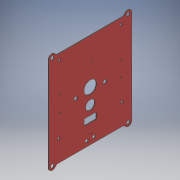
# Autodesk Inventor part: +XPanel_PCB
Saved by Autodesk Inventor 2018 (Build 220112000, 112)
## iProperties
Created: 2018-10-25
Part Number: +XPanel_PCB
Material: Epoxy Resin
Document SubType Name: Modeling
Designer: Bradley
Density: 1.14 g/cm^3
Appearance: Smooth - Dark Gray
Author: Bradley
Autodesk Inventor part; units mm, degrees
ref_plane "YZ Plane" through (0, 0, 0) normal (1, 0, 0) x (0, 1, 0)
ref_plane "XZ Plane" through (0, 0, 0) normal (0, 1, 0) x (-1, 0, 0)
ref_plane "XY Plane" through (0, 0, 0) normal (0, 0, 1) x (1, 0, 0)
sketch "Sketch1" plane through (0, 0, 0) normal (1, 0, 0) x (0, 1, 0)
  line L0 (36.5, -45) -> (-36.5, -45) construction
  line L1 (-36.5, -45) -> (-36.5, 45) construction
  line L2 (-36.5, 45) -> (36.5, 45) construction
  line L3 (36.5, 45) -> (36.5, -45) construction
  line L4 (36.5, -45) -> (-36.5, 45) construction
  line L5 (-36.5, -45) -> (36.5, 45) construction
  line L6 (-14, 0) -> (14, 0) construction
  line L7 (-40, -45) -> (-40, 45)
  arc A0 (-34.0251, 47.4749) -> (-40, 45) centre (-36.5, 45) ccw
  line L8 (-34.0251, 47.4749) -> (-32.3431, 45.7929)
  arc A1 (-32.3431, 45.7929) -> (-31.636, 45.5) centre (-31.636, 46.5) ccw
  line L9 (-31.636, 45.5) -> (31.636, 45.5)
  arc A2 (31.636, 45.5) -> (32.3431, 45.7929) centre (31.636, 46.5) ccw
  line L10 (32.3431, 45.7929) -> (34.0251, 47.4749)
  arc A3 (40, 45) -> (34.0251, 47.4749) centre (36.5, 45) ccw
  line L11 (40, 45) -> (40, -45)
  arc A4 (34.0251, -47.4749) -> (40, -45) centre (36.5, -45) ccw
  line L12 (34.0251, -47.4749) -> (32.3431, -45.7929)
  arc A5 (32.3431, -45.7929) -> (31.636, -45.5) centre (31.636, -46.5) ccw
  line L13 (31.636, -45.5) -> (-31.636, -45.5)
  arc A6 (-31.636, -45.5) -> (-32.3431, -45.7929) centre (-31.636, -46.5) ccw
  line L14 (-32.3431, -45.7929) -> (-34.0251, -47.4749)
  arc A7 (-40, -45) -> (-34.0251, -47.4749) centre (-36.5, -45) ccw
  point P0 (0, 0)
  point P1 (0, 0)
  dimension "d0" = 73
  dimension "d1" = 90
  dimension "d2" = 28
  dimension "d3" = 80
  dimension "d4" = 91
  dimension "d5" = 1
  constraints: 30 end point, 16 point on circle, 16 tangent, 8 centre point, 7 perpendicular, 4 coincident, 4 equal radius, 4 midpoint, 4 parallel, 2 horizontal, 1 vertical
  measures "d0" distance of L1.end L2.end
  measures "d1" distance of L0.end L1.end
  measures "d2" distance of L6.start L6.end
  measures "d3" distance between parallel lines of L11 L7
  measures "d4" distance between parallel lines of L13 L9
  measures "d5" radius of A1
extrude "Extrusion1" add sketch "Sketch1" along normal mid plane 0.6
sketch "Sketch2" plane through (0.3, 0, 0) normal (1, 0, 0) x (0, 0, -1)
  point P0 (0, 0)
  point P1 (-45, -36.5)
  point P2 (-45, 36.5)
  point P3 (0, 14)
  point P4 (0, -14)
  point P5 (45, -36.5)
  point P6 (45, 36.5)
hole "Hole1" at (0.3, -36.5, 45) at (0.3, 36.5, 45) at (0.3, 14, 0) at (0.3, -14, 0) at (0.3, -36.5, -45) at (0.3, 36.5, -45) direction (-1, 0, 0) diameter 3.3 end through all clearance for "Flat Head Machine Screw" size "M3" standard "Ansi Metric M Profile"
sketch "Sketch3" plane through (0.3, 0, 0) normal (1, 0, 0) x (0, 0, -1)
  circle A0 centre (-2.5, 0) radius 6
  circle A1 centre (12.35, 0) radius 4.5
  line L0 (26, -6) -> (22, -6)
  line L1 (21, -5) -> (21, 5)
  line L2 (22, 6) -> (26, 6)
  line L3 (27, 5) -> (27, -5)
  line L4 (27, -6) -> (21, 6) construction
  line L5 (21, -6) -> (27, 6) construction
  arc A2 (21, -5) -> (22, -6) centre (22, -5) ccw
  arc A3 (26, -6) -> (27, -5) centre (26, -5) ccw
  arc A4 (27, 5) -> (26, 6) centre (26, 5) ccw
  arc A5 (22, 6) -> (21, 5) centre (22, 5) ccw
  point P0 (0, 0)
  point P1 (24, 0)
  point P2 (24, 0)
  dimension "d15" = 2.5
  dimension "d16" = 12
  dimension "d17" = 14.85
  dimension "d18" = 9
  dimension "d84" = 24
  dimension "d85" = 12
  dimension "d86" = 6
  dimension "d87" = 1
  constraints: 12 end point, 8 point on circle, 8 point on line, 8 tangent, 6 centre point, 3 equal radius, 3 horizontal alignment, 3 midpoint, 2 parallel, 1 horizontal, 1 perpendicular
  measures "d15" distance of point (0, 0) A0.centre
  measures "d16" diameter of A0
  measures "d17" distance of A1.centre A0.centre
  measures "d18" diameter of A1
  measures "d84" distance of point (0, 0) point (24, 0)
  measures "d85" distance of L5.start L4.end
  measures "d86" distance of L4.start L5.start
  measures "d87" radius of A2
extrude "Extrusion2" cut sketch "Sketch3" against normal through all
sketch "Sketch4" plane through (0.3, 0, 0) normal (1, 0, 0) x (0, 0, -1)
  line L0 (37, -40) -> (38, -40) construction
  line L1 (38, -40) -> (38, 40) construction
  line L2 (38, 40) -> (37, 40) construction
  line L3 (37, 40) -> (37, -40) construction
  line L4 (-11, -40) -> (-10, -40) construction
  line L5 (-10, -40) -> (-10, 40) construction
  line L6 (-10, 40) -> (-11, 40) construction
  line L7 (-11, 40) -> (-11, -40) construction
  circle A0 centre (12.35, 0) radius 4.5 projected
  circle A1 centre (-2.5, 0) radius 6 projected
  circle A2 centre (45, -36.5) radius 1.65 projected
  circle A3 centre (0, 14) radius 1.65 projected
  circle A4 centre (-45, -36.5) radius 1.65 projected
  circle A5 centre (-45, 36.5) radius 1.65 projected
  circle A6 centre (0, -14) radius 1.65 projected
  circle A7 centre (45, 36.5) radius 1.65 projected
  line L8 (-45, -40) -> (45, -40) projected
  arc A8 (45, -40) -> (47.4749, -34.0251) centre (45, -36.5) ccw projected
  line L9 (47.4749, -34.0251) -> (45.7929, -32.3431) projected
  arc A9 (45.5, -31.636) -> (45.7929, -32.3431) centre (46.5, -31.636) ccw projected
  line L10 (45.5, -31.636) -> (45.5, 31.636) projected
  arc A10 (45.7929, 32.3431) -> (45.5, 31.636) centre (46.5, 31.636) ccw projected
  line L11 (45.7929, 32.3431) -> (47.4749, 34.0251) projected
  arc A11 (47.4749, 34.0251) -> (45, 40) centre (45, 36.5) ccw projected
  line L12 (45, 40) -> (-45, 40) projected
  arc A12 (-45, 40) -> (-47.4749, 34.0251) centre (-45, 36.5) ccw projected
  line L13 (-47.4749, 34.0251) -> (-45.7929, 32.3431) projected
  arc A13 (-45.5, 31.636) -> (-45.7929, 32.3431) centre (-46.5, 31.636) ccw projected
  line L14 (-45.5, 31.636) -> (-45.5, -31.636) projected
  arc A14 (-45.7929, -32.3431) -> (-45.5, -31.636) centre (-46.5, -31.636) ccw projected
  line L15 (-45.7929, -32.3431) -> (-47.4749, -34.0251) projected
  arc A15 (-47.4749, -34.0251) -> (-45, -40) centre (-45, -36.5) ccw projected
  line L16 (-20, -40) -> (-19, -40) construction
  line L17 (-19, -40) -> (-19, 40) construction
  line L18 (-20, 40) -> (-20, -40) construction
  line L19 (-19, 40) -> (-20, 40) construction
  line L20 (28, -40) -> (29, -40) construction
  line L21 (29, -40) -> (29, 40) construction
  line L22 (29, 40) -> (28, 40) construction
  line L23 (28, 40) -> (28, -40) construction
  line L24 (-29, -40) -> (-28, -40) construction
  line L25 (-28, -40) -> (-28, 40) construction
  line L26 (-29, 40) -> (-29, -40) construction
  line L27 (-28, 40) -> (-29, 40) construction
  line L28 (19, -40) -> (20, -40) construction
  line L29 (20, -40) -> (20, 40) construction
  line L30 (20, 40) -> (19, 40) construction
  line L31 (19, 40) -> (19, -40) construction
  line L32 (-38, -40) -> (-37, -40) construction
  line L33 (-37, -40) -> (-37, 40) construction
  line L34 (-38, 40) -> (-38, -40) construction
  line L35 (-37, 40) -> (-38, 40) construction
  line L36 (10, -40) -> (11, -40) construction
  line L37 (11, -40) -> (11, 40) construction
  line L38 (11, 40) -> (10, 40) construction
  line L39 (10, 40) -> (10, -40) construction
  line L40 (-10, 0) -> (10, 0) construction
  line L41 (36, -1) -> (36, 1) construction
  circle A16 centre (36, -1) radius 0.75 construction
  circle A17 centre (36, 1) radius 0.75 construction
  circle A18 centre (36, -1) radius 0.35
  circle A19 centre (36, 1) radius 0.35
  line L42 (-38, -13) -> (-12, -13) construction
  line L43 (-12, -13) -> (-12, 13) construction
  line L44 (-12, 13) -> (-38, 13) construction
  line L45 (-38, 13) -> (-38, -13) construction
  circle A20 centre (-23.25, 1.75) radius 0.475
  line L46 (40.5, -3.5) -> (40.5, 3.5) construction
  circle A21 centre (40.5, -3.5) radius 2.25 construction
  circle A22 centre (40.5, 3.5) radius 2.25 construction
  circle A23 centre (28.65, -7) radius 7 construction
  circle A24 centre (21.3666, -25) radius 7 construction
  circle A25 centre (-35.4038, -25) radius 7 construction
  line L47 (35.1389, -9.6256) -> (27.8556, -27.6256) construction
  line L48 (21.3666, -32) -> (-35.4038, -32) construction
  circle A26 centre (25, -30.3897) radius 1 construction
  line L49 (21.3666, -25) -> (25, -30.3897) construction
  arc A27 (21.3666, -32) -> (27.8556, -27.6256) centre (21.3666, -25) ccw construction
  arc A28 (-42.4038, -25) -> (-35.4038, -32) centre (-35.4038, -25) ccw construction
  line L50 (-35.4038, -25) -> (-40, -29.5962) construction
  circle A29 centre (-40, -29.5962) radius 1 construction
  line L51 (35.65, -7) -> (35.65, -1.6633) construction
  line L52 (-42.4038, -25) -> (-42.4038, 0) construction
  line L53 (-45.5, 0) -> (45.5, 0) construction
  line L54 (21.3666, 25) -> (25, 30.3897) construction
  line L55 (-35.4038, 25) -> (-40, 29.5962) construction
  point P0 (36, 0)
  point P1 (0, 0)
  point P2 (-12, 0)
  point P3 (-25, -13)
  point P4 (-38, 0)
  point P5 (-25, 0)
  point P6 (40.5, 0)
  point P7 (25.2795, -30.8043)
  point P8 (-40.3536, -29.9497)
  dimension "d35" = 1.5
  dimension "d25" = 9
  dimension "d30" = 21
  dimension "d31" = 1
  dimension "d34" = 2
  dimension "d38" = 0.7
  dimension "d45" = 26
  dimension "d46" = 12
  dimension "d48" = 0.95
  dimension "d73" = 4.5
  dimension "d74" = 7
  dimension "d75" = 4.5
  dimension "d76" = 40.5
  dimension "d88" = 1.75
  dimension "d89" = 1.75
  dimension "d90" = 14
  dimension "d91" = 7
  dimension "d92" = 7.35
  dimension "d93" = 2
  dimension "d94" = 6.5
  dimension "d96" = 22.03
  dimension "d97" = 32
  dimension "d98" = 40
  dimension "d99" = 25
  constraints: 96 end point, 13 centre point, 12 point on circle, 11 coincident, 10 midpoint, 7 parallel, 7 tangent, 6 point on line, 6 symmetric about line, 5 equal radius, 5 horizontal, 5 horizontal alignment, 3 collinear, 3 equal length, 3 perpendicular, 3 vertical, 1 concentric, 1 vertical alignment, 52 other
  measures "d25" distance of L4.start L16.start
  measures "d30" distance between parallel lines of L37 L5
  measures "d31" distance between parallel lines of L1 L3
  measures "d34" distance of L41.start L41.end
  measures "d38" diameter of A18
  measures "d45" distance of L44.end L43.end
  measures "d46" distance from line of point (0, 0) L43
  measures "d48" diameter of A20
  measures "d73" distance between parallel lines of L46 L41
  measures "d74" distance of L46.start L46.end
  measures "d75" diameter of A21
  measures "d76" distance from line of point (0, 0) L46
  measures "d88" horizontal distance of A20.centre point (-25, 0)
  measures "d89" horizontal distance of A20.centre point (-25, 0)
  measures "d90" diameter of A23
  measures "d91" vertical distance of point (36, 0) A23.centre
  measures "d92" horizontal distance of point (36, 0) A23.centre
  measures "d93" diameter of A26
  measures "d94" distance of L49.start L49.end
  measures "d97" distance from line of A1.centre L48
  measures "d98" horizontal distance of point (0, 0) point (-40, -29.596)
  measures "d99" horizontal distance of point (0, 0) point (25, -30.39)
extrude "Extrusion3" cut sketch "Sketch4" against normal through all contours A18 | A19 | A20
hole "Hole4" at (0.3, -3.5, -40.5) at (0.3, 3.5, -40.5) direction (-1, 0, 0) diameter 3 end through all
hole "Hole5" at (0.3, -30.3897, -25) at (0.3, -29.5962, 40) at (0.3, 30.3897, -25) at (0.3, 29.5962, 40) direction (-1, 0, 0) diameter 2.2 end through all
sketch "Sketch5" plane through (0.3, 0, 0) normal (1, 0, 0) x (0, 0, -1)
  circle A0 centre (25, 30.3897) radius 1.1 projected
  circle A1 centre (25, -30.3897) radius 1.1 projected
  circle A2 centre (-40, -29.5962) radius 1.1 projected
  circle A3 centre (-40, 29.5962) radius 1.1 projected
  circle A4 centre (40.5, -3.5) radius 1.5 projected
  circle A5 centre (40.5, 3.5) radius 1.5 projected
  circle A6 centre (36, -1) radius 0.35 projected
  circle A7 centre (-23.25, 1.75) radius 0.475 projected
  circle A8 centre (36, 1) radius 0.35 projected
  circle A9 centre (12.35, 0) radius 4.5 projected
  circle A10 centre (-2.5, 0) radius 6 projected
  arc A11 (26, -6) -> (27, -5) centre (26, -5) ccw projected
  line L0 (26, -6) -> (22, -6) projected
  arc A12 (21, -5) -> (22, -6) centre (22, -5) ccw projected
  line L1 (21, -5) -> (21, 5) projected
  arc A13 (22, 6) -> (21, 5) centre (22, 5) ccw projected
  line L2 (22, 6) -> (26, 6) projected
  arc A14 (27, 5) -> (26, 6) centre (26, 5) ccw projected
  line L3 (27, 5) -> (27, -5) projected
  circle A15 centre (45, -36.5) radius 1.65 projected
  circle A16 centre (0, 14) radius 1.65 projected
  circle A17 centre (-45, -36.5) radius 1.65 projected
  circle A18 centre (-45, 36.5) radius 1.65 projected
  circle A19 centre (0, -14) radius 1.65 projected
  circle A20 centre (45, 36.5) radius 1.65 projected
  line L4 (-45, -40) -> (45, -40) projected
  arc A21 (45, -40) -> (47.4749, -34.0251) centre (45, -36.5) ccw projected
  line L5 (47.4749, -34.0251) -> (45.7929, -32.3431) projected
  arc A22 (45.5, -31.636) -> (45.7929, -32.3431) centre (46.5, -31.636) ccw projected
  line L6 (45.5, -31.636) -> (45.5, 31.636) projected
  arc A23 (45.7929, 32.3431) -> (45.5, 31.636) centre (46.5, 31.636) ccw projected
  line L7 (45.7929, 32.3431) -> (47.4749, 34.0251) projected
  arc A24 (47.4749, 34.0251) -> (45, 40) centre (45, 36.5) ccw projected
  line L8 (45, 40) -> (-45, 40) projected
  arc A25 (-45, 40) -> (-47.4749, 34.0251) centre (-45, 36.5) ccw projected
  line L9 (-47.4749, 34.0251) -> (-45.7929, 32.3431) projected
  arc A26 (-45.5, 31.636) -> (-45.7929, 32.3431) centre (-46.5, 31.636) ccw projected
  line L10 (-45.5, 31.636) -> (-45.5, -31.636) projected
  arc A27 (-45.7929, -32.3431) -> (-45.5, -31.636) centre (-46.5, -31.636) ccw projected
  line L11 (-45.7929, -32.3431) -> (-47.4749, -34.0251) projected
  arc A28 (-47.4749, -34.0251) -> (-45, -40) centre (-45, -36.5) ccw projected
  line L12 (-11, -29.5) -> (4, -29.5) construction
  line L13 (4, -29.5) -> (4, 29.5) construction
  line L14 (4, 29.5) -> (-11, 29.5) construction
  line L15 (-11, 29.5) -> (-11, -29.5) construction
  line L16 (-12, -13) -> (-12, 13) construction
  point P0 (0, 0)
  point P1 (-11, 0)
  dimension "d107" = 29.5
  dimension "d108" = 15
  dimension "d109" = 1
  constraints: 8 end point, 4 coincident, 2 parallel, 1 horizontal, 1 horizontal alignment, 1 midpoint, 1 perpendicular
  measures "d107" distance from line of A10.centre L12
  measures "d108" distance of L12.start L12.end
  measures "d109" distance between parallel lines of L15 L16
hole "Hole6" at (0.3, -29.5, 11) at (0.3, -29.5, -4) at (0.3, 29.5, -4) at (0.3, 29.5, 11) direction (-1, 0, 0) diameter 1 end through all
body "Solid1"
